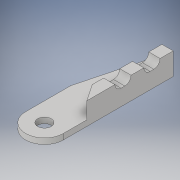
# Autodesk Inventor part: chain_end_elmt
Saved by Autodesk Inventor 2019.3 (Build 233278000, 278)
## iProperties
Created: 2020-08-28
Part Number: chain_end_elmt
Material: Generisch
Document SubType Name: Modeling
Designer: Nicolas Frick
Density: 1 g/cm^3
Appearance: Vorgabe
Author: Nicolas Frick
Autodesk Inventor part; units mm, degrees
ref_plane "YZ Plane" through (0, 0, 0) normal (1, 0, 0) x (0, 1, 0)
ref_plane "XZ Plane" through (0, 0, 0) normal (0, 1, 0) x (-1, 0, 0)
ref_plane "XY Plane" through (0, 0, 0) normal (0, 0, 1) x (1, 0, 0)
sketch "Skizze1" plane through (0, 0, 0) normal (0, 1, 0) x (-1, 0, 0)
  arc A0 (5, 0) -> (-5, 0) centre (0, 0) ccw
  circle A1 centre (0, 0) radius 1.8
  line L0 (-5, 0) -> (-5, -29.2)
  line L1 (-5, -29.2) -> (0.5, -29.2)
  line L2 (5, 0) -> (5, -12)
  line L3 (5, -12) -> (0.5, -29.2)
  dimension "d0" = 10
  dimension "d1" = 3.6
  dimension "d2" = 29.2
  dimension "d3" = 5.5
  dimension "d4" = 12
  constraints: 8 end point, 2 centre point, 2 coincident, 2 point on circle, 2 vertical, 1 perpendicular
  measures "d0" diameter of A0
  measures "d1" diameter of A1
  measures "d2" distance of L0.start L0.end
  measures "d3" distance of L0.end L1.end
  measures "d4" distance of L2.start L2.end
extrude "Extrusion1" add sketch "Skizze1" along normal blind 1.5
sketch "Skizze2" plane through (0, 1.5, 0) normal (0, 1, 0) x (1, 0, 0)
  line L0 (4.9805, 29.2565) -> (5, 6.2565)
  line L1 (5, 0) -> (5, 29.2) projected
  line L2 (5, 29.2) -> (2, 29.2)
  line L3 (2, 29.2) -> (2, 10.7)
  line L4 (2, 10.7) -> (5, 6.2565)
  point P0 (0, 0)
  dimension "d7" = 23
  dimension "d8" = 3
  dimension "d9" = 18.5
  constraints: 8 end point, 1 horizontal, 1 perpendicular, 1 point on line
  measures "d7" distance of L0.start L0.end
  measures "d8" distance of L1.end L2.end
  measures "d9" distance of L2.end L3.end
extrude "Extrusion2" add sketch "Skizze2" along normal blind 4.4
sketch "Skizze3" plane through (2, 1.5, -29.2) normal (-1, 0, 0) x (0, 0, 1)
  line L0 (22.9435, 4.4) -> (0, 4.4) construction
  line L1 (0, 4.4) -> (3.5, 4.4) construction
  line L2 (0, 3.6562) -> (11.2, 3.6562) construction
  line L3 (3.5, 4.4) -> (7.8, 4.4) construction
  line L4 (11.2, 4.4) -> (15.5, 4.4) construction
  line L5 (3.5, 4.4) -> (7.8, 4.4) construction
  line L6 (5.15, 2.75) -> (6.15, 2.75)
  arc A0 (3.5, 4.4) -> (5.15, 2.75) centre (5.15, 4.4) ccw
  arc A1 (6.15, 2.75) -> (7.8, 4.4) centre (6.15, 4.4) ccw
  line L7 (11.2, 4.4) -> (15.5, 4.4) construction
  line L8 (12.85, 2.75) -> (13.85, 2.75)
  arc A2 (11.2, 4.4) -> (12.85, 2.75) centre (12.85, 4.4) ccw
  arc A3 (13.85, 2.75) -> (15.5, 4.4) centre (13.85, 4.4) ccw
  line L9 (3.5, 4.4) -> (7.8, 4.4)
  line L10 (11.2, 4.4) -> (15.5, 4.4)
  point P0 (29.2, -1.5)
  point P1 (5.65, 4.4)
  point P2 (13.35, 4.4)
  constraints: 24 end point, 12 point on circle, 8 point on line, 4 centre point, 4 collinear, 4 tangent, 2 midpoint, 1 horizontal
extrude "Extrusion3" cut sketch "Skizze3" against normal blind 4.4
